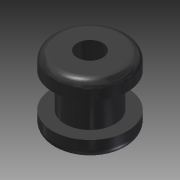
# Autodesk Inventor part: Grommet
Saved by Autodesk Inventor 2015 (Build 190159000, 159)
## iProperties
Created: 2014-03-05
Part Number: Grommet
Material: Generic
Document SubType Name: Modeling
Designer: Jonathan
Density: 1 g/cm^3
Appearance: Default
Author: Jonathan
Autodesk Inventor part; units mm, degrees
ref_plane "YZ Plane" through (0, 0, 0) normal (1, 0, 0) x (0, 1, 0)
ref_plane "XZ Plane" through (0, 0, 0) normal (0, 1, 0) x (-1, 0, 0)
ref_plane "XY Plane" through (0, 0, 0) normal (0, 0, 1) x (1, 0, 0)
sketch "Sketch1" plane through (0, 0, 0) normal (0, 0, 1) x (1, 0, 0)
  line L0 (1.5, 0) -> (1.5, 4.05)
  line L1 (1.5, 4.05) -> (4.4, 4.05)
  line L2 (4.4, 4.05) -> (4.4, 2)
  line L3 (4.4, 2) -> (2.95, 2)
  line L4 (2.95, 2) -> (2.95, 0)
  line L5 (0, 0) -> (18.7234, 0) construction
  line L6 (0, 16.7698) -> (0, -15.2532)
  line L7 (1.5, 0) -> (1.5, -4.05)
  line L8 (1.5, -4.05) -> (4.4, -4.05)
  line L9 (4.4, -4.05) -> (4.4, -2)
  line L10 (4.4, -2) -> (2.95, -2)
  line L11 (2.95, -2) -> (2.95, 0)
  dimension "d1" = 0
  dimension "d3" = 3
  dimension "d4" = 5.9
  dimension "d5" = 8.8
  dimension "d6" = 8.1
  dimension "d7" = 4
  constraints: 24 end point, 4 symmetric about line, 3 parallel, 3 perpendicular, 1 vertical
  measures "d1" distance from line of L5.start L6
  measures "d3" diameter of L0 L6
  measures "d4" diameter of L4 L6
  measures "d5" diameter of L2 L6
  measures "d6" distance between parallel lines of L8 L1
  measures "d7" distance between parallel lines of L10 L3
revolve "Revolution1" add sketch "Sketch1" angle 360 about axis through (0, 16.7698, 0) along (0, -1, 0)
fillet "Fillet1" radius 1 1 edges at (-4.4, 4.05, 0)
fillet "Fillet2" radius 1 1 edges at (-4.4, -4.05, 0)
body "Solid1"
